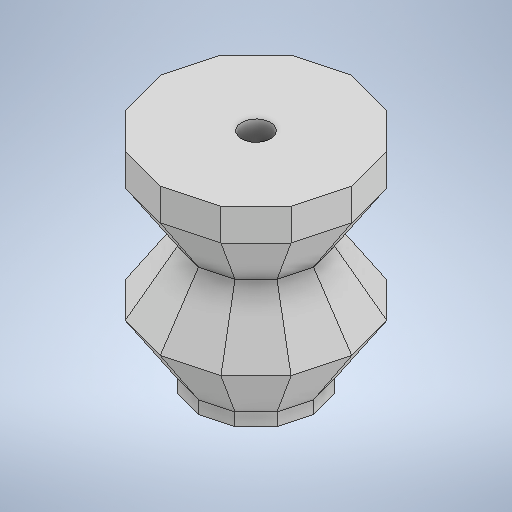
# Autodesk Inventor part: diameter30mm
Saved by Autodesk Inventor 2025.1 (Build 291241000, 241)
## iProperties
Created: 2024-08-08
Part Number: diameter30mm
Material: 일반
Document SubType Name: Modeling
Designer: 82103
Density: 1 g/cm^3
Appearance: 기본값
Author: 82103
Autodesk Inventor part; units mm, degrees
ref_plane "YZ Plane" through (0, 0, 0) normal (1, 0, 0) x (0, 1, 0)
ref_plane "XY Plane" through (0, 0, 0) normal (0, 0, 1) x (1, 0, 0)
sketch "스케치1" plane through (0, 0, 0) normal (0, 1, 0) x (-1, 0, 0)
  line L0 (12.9904, -7.5) -> (7.5, -12.9904)
  line L1 (7.5, -12.9904) -> (0, -15)
  line L2 (0, -15) -> (-7.5, -12.9904)
  line L3 (-7.5, -12.9904) -> (-12.9904, -7.5)
  line L4 (-12.9904, -7.5) -> (-15, 0)
  line L5 (-15, 0) -> (-12.9904, 7.5)
  line L6 (-12.9904, 7.5) -> (-7.5, 12.9904)
  line L7 (-7.5, 12.9904) -> (0, 15)
  line L8 (0, 15) -> (7.5, 12.9904)
  line L9 (7.5, 12.9904) -> (12.9904, 7.5)
  line L10 (12.9904, 7.5) -> (15, 0)
  line L11 (15, 0) -> (12.9904, -7.5)
  point P0 (0, 0)
  point P1 (0, 0)
  dimension "d0" = 30
  constraints: 24 end point, 1 coincident, 1 horizontal alignment, 25 other
  measures "d0" distance of L4.end L10.end
ref_plane "작업 평면1" through (0, 9, 0) normal (0, 1, 0) x (-1, 0, 0)
sketch "스케치2" plane through (0, 9, 0) normal (0, 1, 0) x (-1, 0, 0)
  line L0 (7.7942, -4.5) -> (4.5, -7.7942)
  line L1 (4.5, -7.7942) -> (0, -9)
  line L2 (0, -9) -> (-4.5, -7.7942)
  line L3 (-4.5, -7.7942) -> (-7.7942, -4.5)
  line L4 (-7.7942, -4.5) -> (-9, 0)
  line L5 (-9, 0) -> (-7.7942, 4.5)
  line L6 (-7.7942, 4.5) -> (-4.5, 7.7942)
  line L7 (-4.5, 7.7942) -> (0, 9)
  line L8 (0, 9) -> (4.5, 7.7942)
  line L9 (4.5, 7.7942) -> (7.7942, 4.5)
  line L10 (7.7942, 4.5) -> (9, 0)
  line L11 (9, 0) -> (7.7942, -4.5)
  point P0 (0, 0)
  point P1 (0, 0)
  dimension "d2" = 18
  constraints: 24 end point, 1 coincident, 1 horizontal alignment, 25 other
  measures "d2" distance of L4.end L10.end
loft "로프트1" add profiles "스케치2", "스케치1"
mirror "미러1" about plane through (0, 9, 0) normal (0, 1, 0) of "로프트1"
mirror "미러2" about plane through (0, 0, 0) normal (0, 1, 0) of "로프트1"
shell "쉘1" thickness 0.5 removed faces 0 ; own thickness 2 on faces at (3.5, -1.5, 13.0622) (9.5622, -1.5, 9.5622) (13.0622, -1.5, 3.5) (13.0622, -1.5, -3.5) (9.5622, -1.5, -9.5622) (3.5, -1.5, -13.0622) (-3.5, -1.5, -13.0622) (-9.5622, -1.5, -9.5622) (-13.0622, -1.5, -3.5) (-13.0622, -1.5, 3.5) (-9.5622, -1.5, 9.5622) (-3.5, -1.5, 13.0622) (-3.5, 16.5, -13.0622) (-9.5622, 16.5, -9.5622) (-13.0622, 16.5, -3.5) (-13.0622, 16.5, 3.5) (-9.5622, 16.5, 9.5622) (-3.5, 16.5, 13.0622) (3.5, 16.5, 13.0622) (9.5622, 16.5, 9.5622) (13.0622, 16.5, 3.5) (13.0622, 16.5, -3.5) (9.5622, 16.5, -9.5622) (3.5, 16.5, -13.0622)
sketch "스케치3" plane through (0, 0, 0) normal (1, 0, 0) x (0, 1, 0)
  point P0 (0, 0)
sketch "스케치4" plane through (-4.5, -9, -7.7942) normal (0, -1, 0) x (0.7071068, 0, 0.7071068)
  line L0 (11.0227, 11.0227) -> (6.364, 11.0227) projected
  line L1 (15.0573, 8.6933) -> (11.0227, 11.0227) projected
  line L2 (17.3867, 4.6587) -> (15.0573, 8.6933) projected
  line L3 (17.3867, 0) -> (17.3867, 4.6587) projected
  line L4 (15.0573, -4.0346) -> (17.3867, 0) projected
  line L5 (11.0227, -6.364) -> (15.0573, -4.0346) projected
  line L6 (6.364, -6.364) -> (11.0227, -6.364) projected
  line L7 (2.3294, -4.0346) -> (6.364, -6.364) projected
  line L8 (0, 0) -> (2.3294, -4.0346) projected
  line L9 (0, 4.6587) -> (0, 0) projected
  line L10 (2.3294, 8.6933) -> (0, 4.6587) projected
  line L11 (6.364, 11.0227) -> (2.3294, 8.6933) projected
  point P0 (8.6933, 2.3294)
extrude "돌출1" add sketch "스케치4" along normal blind 2
sketch "스케치5" plane through (-12.9904, 18, -7.5) normal (0, 1, 0) x (0.7071068, 0, 0.7071068)
  line L0 (10.6066, 18.3712) -> (18.3712, 18.3712) projected
  line L1 (18.3712, 18.3712) -> (25.0955, 14.4889) projected
  line L2 (25.0955, 14.4889) -> (28.9778, 7.7646) projected
  line L3 (28.9778, 7.7646) -> (28.9778, 0) projected
  line L4 (28.9778, 0) -> (25.0955, -6.7243) projected
  line L5 (25.0955, -6.7243) -> (18.3712, -10.6066) projected
  line L6 (18.3712, -10.6066) -> (10.6066, -10.6066) projected
  line L7 (10.6066, -10.6066) -> (3.8823, -6.7243) projected
  line L8 (3.8823, -6.7243) -> (0, 0) projected
  line L9 (0, 0) -> (0, 7.7646) projected
  line L10 (0, 7.7646) -> (3.8823, 14.4889) projected
  line L11 (3.8823, 14.4889) -> (10.6066, 18.3712) projected
  point P0 (14.4889, 3.8823)
sketch "스케치6" plane through (-12.9904, 18, -7.5) normal (0, 1, 0) x (0.7071068, 0, 0.7071068)
  point P0 (14.4889, 3.8823)
extrude "돌출2" add sketch "스케치5" along normal blind 5
sketch "스케치7" plane through (-12.9904, 23, -7.5) normal (0, 1, 0) x (0.7071068, 0, -0.7071068)
  circle A0 centre (3.8823, -14.4889) radius 2.25
  dimension "d13" = 4.5
  constraints: 1 centre point, 1 coincident
  measures "d13" diameter of A0
extrude "돌출3" cut sketch "스케치7" against normal blind 5.5
sketch "스케치8" plane through (0, 0, 0) normal (0, 0, 1) x (1, 0, 0)
  point P0 (0, 0)
ref_plane "작업 평면2" through (0, 0, 0) normal (0, 1, 0) x (-1, 0, 0)
